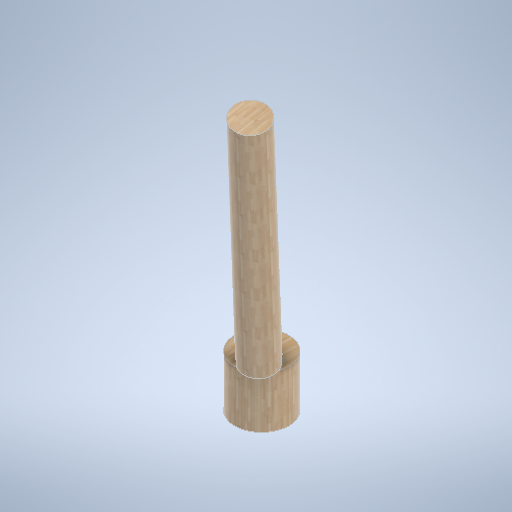
# Autodesk Inventor part: Maple_Tree
Saved by Autodesk Inventor 2025 (Build 290162010, 162A)
## iProperties
Created: 2024-08-07
Part Number: Maple_Tree
Material: Wood (Maple)
Document SubType Name: Modeling
Designer: Tom
Density: 0.67 g/cm^3
Appearance: Natural Maple - Glossy Dark Tint
Author: Tom
Autodesk Inventor part; units mm, degrees
ref_plane "YZ Plane" through (0, 0, 0) normal (1, 0, 0) x (0, 1, 0)
sketch "Sketch1" plane through (0, 0, 0) normal (0, 1, 0) x (-1, 0, 0)
  circle A0 centre (0, 0) radius 635
  dimension "d0" = 1270
  constraints: 1 centre point, 1 coincident
  measures "d0" diameter of A0
extrude "Extrusion1" add sketch "Sketch1" along normal blind 1219.2
ref_plane "Work Plane2" through (0, 0, 635) normal (0, 0, 1) x (1, 0, 0)
ref_plane "Work Plane3" through (0, 0, 939.8) normal (0, 0, 1) x (1, 0, 0)
sketch "Sketch2" plane through (0, 1219.2, 0) normal (0, 1, 0) x (1, 0, 0)
  line L0 (0, 0) -> (698.5, -863.6)
  line L1 (698.5, -863.6) -> (0, -863.6)
  line L2 (0, -863.6) -> (0, 0)
  circle A0 centre (0, 0) radius 635 projected
  line L3 (1039.1588, -635) -> (-914.0265, -635) projected
  line L4 (1039.1588, -939.8) -> (-914.0265, -939.8) projected
  line L5 (760.1324, -939.8) -> (0, -939.8)
  point P0 (513.6029, -635)
  dimension "d3" = 863.6
  dimension "d11" = 698.5
  constraints: 8 end point, 4 point on line, 1 horizontal, 1 vertical
  measures "d3" distance of L1.end L0.start
  measures "d11" distance of L0.end L1.end
ref_plane "Work Plane5" through (0, 1219.2, 0) normal (-0.7775111, 0, 0.6288692) x (0.6288692, 0, 0.7775111)
sketch "Sketch4" plane through (0, 1219.2, 0) normal (0, 1, 0) x (1, 0, 0)
  line L0 (0, -863.6) -> (0, 0) projected
  line L1 (1024.4813, -1266.6315) -> (-825.9616, 1021.1889) projected
  line L2 (1039.1588, -939.8) -> (-914.0265, -939.8) projected
  line L3 (0, -838.2) -> (677.9559, -838.2)
  dimension "d10" = 101.6
  constraints: 2 end point, 2 point on line, 1 horizontal
  measures "d10" distance between parallel lines of L3 L2
sketch "Sketch3" plane through (0, 1219.2, 0) normal (-0.7775111, 0, 0.6288692) x (0.6288692, 0, 0.7775111)
  line L0 (1208.7288, 0) -> (1208.7288, 1117.6)
  line L1 (635, -1219.2) -> (-635, -1219.2) projected
  line L2 (816.7086, 0) -> (1078.0554, 1117.6)
  line L3 (1078.0554, 0) -> (1078.0554, 1117.6)
  line L4 (0, 0) -> (303.6922, 1298.6821)
  line L5 (1078.0554, 1117.6) -> (303.6922, 1298.6821)
  line L6 (816.7086, 0) -> (42.3454, 181.0821)
  line L7 (429.527, 90.541) -> (1817.6069, 6026.4024)
  line L8 (303.6922, 1298.6821) -> (1430.4253, 6116.9434)
  line L9 (1430.4253, 6116.9434) -> (2204.7886, 5935.8614)
  line L10 (2204.7886, 5935.8614) -> (1078.0554, 1117.6)
  point P0 (0, -1219.2)
  point P1 (690.8738, 1208.141)
  dimension "d8" = 1117.6
  dimension "d9" = 1219.2
  dimension "d13" = 6096
  constraints: 20 end point, 3 midpoint, 3 perpendicular, 2 collinear, 2 parallel, 2 point on line, 2 vertical, 1 coincident
  measures "d8" distance of L0.start L0.end
  measures "d9" distance from line of L1 L2.start
  measures "d13" distance of L7.start L7.end
revolve "Revolution1" add sketch "Sketch3" angle 360 about axis through (270.1163, 1309.741, 333.962) along (0.1431957, 0.9737305, 0.1770419) contours L6 L4 L5 L7 | L5 L8 L9 L7
body "Solid1"
